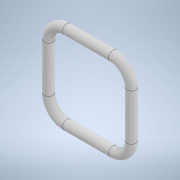
# Autodesk Inventor part: Деталь8
Saved by Autodesk Inventor 2021.1 (Build 251245010, 245A)
## iProperties
Created: 2023-10-24
Part Number: Деталь8
Material: Типовые
Document SubType Name: Modeling
Designer: Lenovo
Density: 1 g/cm^3
Appearance: По умолчанию
Author: Lenovo
Autodesk Inventor part; units mm, degrees
ref_plane "YZ Plane" through (0, 0, 0) normal (1, 0, 0) x (0, 1, 0)
ref_plane "XZ Plane" through (0, 0, 0) normal (0, 1, 0) x (-1, 0, 0)
ref_plane "XY Plane" through (0, 0, 0) normal (0, 0, 1) x (1, 0, 0)
sketch "Эскиз1" plane through (0, 0, 0) normal (0, 1, 0) x (-1, 0, 0)
  circle A0 centre (0, 0) radius 1
  dimension "d0" = 2
  constraints: 1 centre point, 1 coincident
  measures "d0" diameter of A0
sketch "Эскиз2" plane through (0, 0, 0) normal (0, 0, 1) x (1, 0, 0)
  line L0 (0, 0) -> (0, 5)
  line L1 (4, 9) -> (14, 9)
  line L2 (18, 5) -> (18, -5)
  line L3 (14, -9) -> (4, -9)
  line L4 (0, -5) -> (0, 0)
  arc A0 (4, 9) -> (0, 5) centre (4, 5) ccw
  arc A1 (18, 5) -> (14, 9) centre (14, 5) ccw
  arc A2 (14, -9) -> (18, -5) centre (14, -5) ccw
  arc A3 (0, -5) -> (4, -9) centre (4, -5) ccw
  point P0 (0, 9)
  point P1 (18, 9)
  point P2 (18, -9)
  point P3 (0, -9)
  dimension "d1" = 9
  dimension "d2" = 18
  dimension "d3" = 18
  dimension "d4" = 18
  dimension "d5" = 4
  constraints: 10 end point, 9 point on line, 8 point on circle, 8 tangent, 4 centre point, 3 equal radius, 2 perpendicular, 1 collinear, 1 vertical
  measures "d1" distance of L0.start point (0, 9)
  measures "d2" distance of point (0, 9) point (18, 9)
  measures "d3" distance of point (18, 9) point (18, -9)
  measures "d4" distance of point (18, -9) point (0, -9)
  measures "d5" radius of A0
sweep "Сдвиг1" add profiles "Эскиз1" path "Эскиз2"
